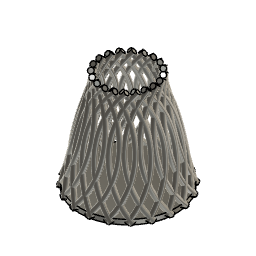
Untitled (Autodesk Fusion 360 design; units mm, degrees)
Autodesk Fusion 360 part; units mm, degrees
sketch "Sketch1" plane through (0, 0, 0) normal (0, 0, 1) x (1, 0, 0)
  circle A0 centre (0, 0) radius 50
  dimension "d1" = 100
  constraint coincident A0.centre origin
  measures "d1" diameter of A0
extrude "Extrude1" add sketch "Sketch1" along normal blind 5 makes body 1
ref_plane "WorkPlane1" through (0, 0, 105) normal (0, 0, 1) x (1, 0, 0)
sketch "Sketch2" plane through (0, 0, 105) normal (0, 0, 1) x (1, 0, 0)
  circle A0 centre (0, 0) radius 25
  dimension "d5" = 50
  constraint coincident A0.centre origin
  measures "d5" diameter of A0
sketch "Sketch3" plane through (0, 0, 0) normal (1, 0, 0) x (0, 1, 0)
sketch "Sketch4" plane through (0, 0, 0) normal (1, 0, 0) x (0, 1, 0)
  line L0 (0, 0) -> (0, 105)
  dimension "d25" = 105
  constraint coincident L0.start origin
  constraint vertical L0
  measures "d25" distance of L0.start L0.end
ref_plane "WorkPlane2" through (50, 0, 0) normal (1, 0, 0) x (0, 1, 0)
sketch "Sketch5" plane through (50, 0, 0) normal (1, 0, 0) x (0, 1, 0)
sketch "Sketch6" plane through (0, 0, 0) normal (0, 1, 0) x (1, 0, 0)
ref_plane "WorkPlane3" through (37.5, 0, 52.5) normal (0.972806, 0, 0.231621) x (-0.231621, 0, 0.972806)
sketch "Sketch10" plane through (37.5, 0, 52.5) normal (0.972806, 0, 0.231621) x (-0.231621, 0, 0.972806)
  arc A0 through (52.2596, -11.5129, -0.4885) (-0.2404, 8.4871, -0.4885) (-52.7404, -11.5129, -0.4885)
  arc A1 through (-52.7404, 8.4871, -0.4885) (-0.2404, -11.5129, -0.4885) (52.2596, 8.4871, -0.4885)
pipe "Pipe1" add diameter 5 path "Sketch10" along A1 separate body makes body 2 in component "Component"
pipe "Pipe1'" add diameter 5 path "Sketch10" along A0 separate body makes body 3 in component "Component'"
component_pattern "component pattern"
component "Component" placed x (1, 0, 0) y (0, 1, 0) z (0, 0, 1) at (0, 0, 0)
component "Component'" placed x (1, 0, 0) y (0, 1, 0) z (0, 0, 1) at (0, 0, 0)
component "Component" placed x (0.951057, 0.309017, 0) y (-0.309017, 0.951057, 0) z (0, 0, 1) at (0, 0, 0)
component "Component'" placed x (0.951057, 0.309017, 0) y (-0.309017, 0.951057, 0) z (0, 0, 1) at (0, 0, 0)
component "Component" placed x (0.809017, 0.587785, 0) y (-0.587785, 0.809017, 0) z (0, 0, 1) at (0, 0, 0)
component "Component'" placed x (0.809017, 0.587785, 0) y (-0.587785, 0.809017, 0) z (0, 0, 1) at (0, 0, 0)
component "Component" placed x (0.587785, 0.809017, 0) y (-0.809017, 0.587785, 0) z (0, 0, 1) at (0, 0, 0)
component "Component'" placed x (0.587785, 0.809017, 0) y (-0.809017, 0.587785, 0) z (0, 0, 1) at (0, 0, 0)
component "Component" placed x (0.309017, 0.951057, 0) y (-0.951057, 0.309017, 0) z (0, 0, 1) at (0, 0, 0)
component "Component'" placed x (0.309017, 0.951057, 0) y (-0.951057, 0.309017, 0) z (0, 0, 1) at (0, 0, 0)
component "Component" placed x (0, 1, 0) y (-1, 0, 0) z (0, 0, 1) at (0, 0, 0)
component "Component'" placed x (0, 1, 0) y (-1, 0, 0) z (0, 0, 1) at (0, 0, 0)
component "Component" placed x (-0.309017, 0.951057, 0) y (-0.951057, -0.309017, 0) z (0, 0, 1) at (0, 0, 0)
component "Component'" placed x (-0.309017, 0.951057, 0) y (-0.951057, -0.309017, 0) z (0, 0, 1) at (0, 0, 0)
component "Component" placed x (-0.587785, 0.809017, 0) y (-0.809017, -0.587785, 0) z (0, 0, 1) at (0, 0, 0)
component "Component'" placed x (-0.587785, 0.809017, 0) y (-0.809017, -0.587785, 0) z (0, 0, 1) at (0, 0, 0)
component "Component" placed x (-0.809017, 0.587785, 0) y (-0.587785, -0.809017, 0) z (0, 0, 1) at (0, 0, 0)
component "Component'" placed x (-0.809017, 0.587785, 0) y (-0.587785, -0.809017, 0) z (0, 0, 1) at (0, 0, 0)
component "Component" placed x (-0.951057, 0.309017, 0) y (-0.309017, -0.951057, 0) z (0, 0, 1) at (0, 0, 0)
component "Component'" placed x (-0.951057, 0.309017, 0) y (-0.309017, -0.951057, 0) z (0, 0, 1) at (0, 0, 0)
component "Component" placed x (-1, 0, 0) y (0, -1, 0) z (0, 0, 1) at (0, 0, 0)
component "Component'" placed x (-1, 0, 0) y (0, -1, 0) z (0, 0, 1) at (0, 0, 0)
component "Component" placed x (-0.951057, -0.309017, 0) y (0.309017, -0.951057, 0) z (0, 0, 1) at (0, 0, 0)
component "Component'" placed x (-0.951057, -0.309017, 0) y (0.309017, -0.951057, 0) z (0, 0, 1) at (0, 0, 0)
component "Component" placed x (-0.809017, -0.587785, 0) y (0.587785, -0.809017, 0) z (0, 0, 1) at (0, 0, 0)
component "Component'" placed x (-0.809017, -0.587785, 0) y (0.587785, -0.809017, 0) z (0, 0, 1) at (0, 0, 0)
component "Component" placed x (-0.587785, -0.809017, 0) y (0.809017, -0.587785, 0) z (0, 0, 1) at (0, 0, 0)
component "Component'" placed x (-0.587785, -0.809017, 0) y (0.809017, -0.587785, 0) z (0, 0, 1) at (0, 0, 0)
component "Component" placed x (-0.309017, -0.951057, 0) y (0.951057, -0.309017, 0) z (0, 0, 1) at (0, 0, 0)
component "Component'" placed x (-0.309017, -0.951057, 0) y (0.951057, -0.309017, 0) z (0, 0, 1) at (0, 0, 0)
component "Component" placed x (0, -1, 0) y (1, 0, 0) z (0, 0, 1) at (0, 0, 0)
component "Component'" placed x (0, -1, 0) y (1, 0, 0) z (0, 0, 1) at (0, 0, 0)
component "Component" placed x (0.309017, -0.951057, 0) y (0.951057, 0.309017, 0) z (0, 0, 1) at (0, 0, 0)
component "Component'" placed x (0.309017, -0.951057, 0) y (0.951057, 0.309017, 0) z (0, 0, 1) at (0, 0, 0)
component "Component" placed x (0.587785, -0.809017, 0) y (0.809017, 0.587785, 0) z (0, 0, 1) at (0, 0, 0)
component "Component'" placed x (0.587785, -0.809017, 0) y (0.809017, 0.587785, 0) z (0, 0, 1) at (0, 0, 0)
component "Component" placed x (0.809017, -0.587785, 0) y (0.587785, 0.809017, 0) z (0, 0, 1) at (0, 0, 0)
component "Component'" placed x (0.809017, -0.587785, 0) y (0.587785, 0.809017, 0) z (0, 0, 1) at (0, 0, 0)
component "Component" placed x (0.951057, -0.309017, 0) y (0.309017, 0.951057, 0) z (0, 0, 1) at (0, 0, 0)
component "Component'" placed x (0.951057, -0.309017, 0) y (0.309017, 0.951057, 0) z (0, 0, 1) at (0, 0, 0)
